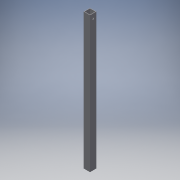
# Autodesk Inventor part: Pivot point Support
Saved by Autodesk Inventor 2017 (Build 210142000, 142)
## iProperties
Created: 2019-01-22
Part Number: Pivot point Support
Material: Generic
Document SubType Name: Modeling
Designer: S346795925
Density: 1 g/cm^3
Appearance: Default
Author: S346795925
Autodesk Inventor part; units mm, degrees
ref_plane "YZ Plane" through (0, 0, 0) normal (1, 0, 0) x (0, 1, 0)
ref_plane "XZ Plane" through (0, 0, 0) normal (0, 1, 0) x (-1, 0, 0)
ref_plane "XY Plane" through (0, 0, 0) normal (0, 0, 1) x (1, 0, 0)
sketch "Sketch1" plane through (0, 0, 0) normal (0, 1, 0) x (-1, 0, 0)
  line L0 (0, 0) -> (-38.1, 0)
  line L1 (-38.1, 0) -> (-38.1, -38.1)
  line L2 (-38.1, -38.1) -> (0, -38.1)
  line L3 (0, -38.1) -> (0, 0)
  line L4 (-3.175, -3.175) -> (-34.925, -3.175)
  line L5 (-34.925, -3.175) -> (-34.925, -34.925)
  line L6 (-34.925, -34.925) -> (-3.175, -34.925)
  line L7 (-3.175, -34.925) -> (-3.175, -3.175)
  dimension "d0" = 38.1
  dimension "d1" = 38.1
  dimension "d2" = 3.175
  constraints: 16 end point, 4 parallel, 2 perpendicular, 1 horizontal, 3 other
  measures "d0" distance of L2.end L1.end
  measures "d1" distance of L1.end L0.end
  measures "d2" distance between parallel lines of L3 L7
extrude "Extrusion1" add sketch "Sketch1" along normal blind 809.625
sketch "Sketch2" plane through (38.1, 0, 0) normal (1, 0, 0) x (0, 0, -1)
  circle A0 centre (19.05, 784.225) radius 6.35
  line L0 (0, 809.625) -> (38.1, 809.625) projected
  point P0 (0, 0)
  dimension "d5" = 12.7
  dimension "d6" = 25.4
  constraints: 1 centre point
  measures "d5" diameter of A0
  measures "d6" distance from line of L0 A0.centre
extrude "Extrusion2" cut sketch "Sketch2" against normal through all
body "Solid1"
